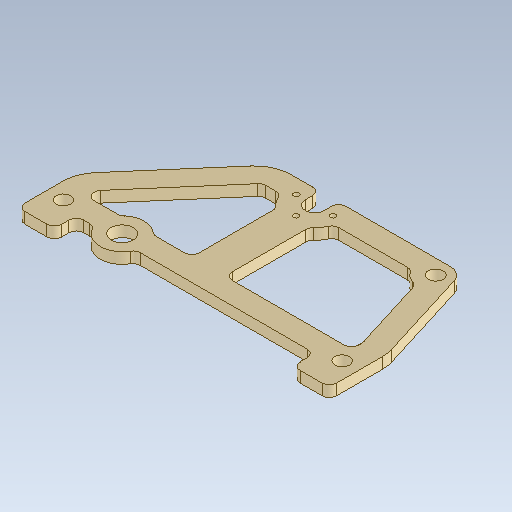
# Autodesk Inventor part: Опора катушки (врунтренняя)
Saved by Autodesk Inventor 2021.1 (Build 251245010, 245A)
## iProperties
Created: 2026-04-13
Part Number: Опора катушки (врунтренняя)
Material: Типовые
Document SubType Name: Modeling
Designer: Андрей Тарасов
Density: 1 g/cm^3
Appearance: По умолчанию
Author: Андрей Тарасов
Autodesk Inventor part; units mm, degrees
ref_plane "YZ Plane" through (0, 0, 0) normal (1, 0, 0) x (0, 1, 0)
ref_plane "XZ Plane" through (0, 0, 0) normal (0, 1, 0) x (-1, 0, 0)
ref_plane "XY Plane" through (0, 0, 0) normal (0, 0, 1) x (1, 0, 0)
sketch "Эскиз1" plane through (0, 0, 0) normal (0, 0, 1) x (1, 0, 0)
  circle A0 centre (0, 0) radius 60 construction
  line L0 (-80, -70) -> (-80, -50)
  line L1 (-80, -50) -> (-30, 8)
  line L2 (-30, 8) -> (72, 8)
  line L3 (72, 8) -> (90, -50)
  line L4 (90, -50) -> (90, -70)
  line L5 (90, -70) -> (-80, -70)
  line L6 (0, -110.4) -> (0, 88.4) construction
  line L7 (-115.4, 0) -> (132.4, 0) construction
  line L8 (-80, -50) -> (90, -50) construction
  circle A1 centre (67, -35) radius 12.5 construction
  circle A2 centre (0, 0) radius 5.1
  circle A3 centre (66, 0) radius 4.1
  circle A4 centre (67, -35) radius 4
  circle A5 centre (67, -35) radius 8.5 construction
  line L9 (67, -49.1463) -> (67, -22.5) construction
  circle A6 centre (67, -43.5) radius 1.6
  circle A7 centre (67, -26.5) radius 1.6
  line L10 (-24.5014, -4) -> (-68, -54.4584)
  line L11 (-68, -54.4584) -> (-68, -58)
  line L12 (-68, -58) -> (78, -58)
  line L13 (78, -58) -> (78, -51.8193)
  line L14 (78, -51.8193) -> (63.1595, -4)
  line L15 (63.1595, -4) -> (-24.5014, -4)
  arc A8 (-3.5925, -14.5634) -> (14.4568, -4) centre (0, 0) ccw
  arc A9 (-14.4568, -4) -> (-3.5925, -14.5634) centre (0, 0) ccw
  arc A10 (14.4568, -4) -> (-14.4568, -4) centre (0, 0) ccw construction
  line L16 (-9, -58) -> (-9, -12)
  line L17 (9, -58) -> (9, -12)
  arc A11 (65.0062, -9.9505) -> (56.8348, -4) centre (66, 0) ccw construction
  line L18 (68.4354, -21) -> (58.4354, -21)
  line L19 (58.4354, -21) -> (47.8258, -58)
  arc A12 (56.8348, -4) -> (65.0062, -9.9505) centre (66, 0) ccw
  line L20 (-80, -70) -> (-80, -82)
  line L21 (-80, -82) -> (-60, -82)
  line L22 (-60, -82) -> (-60, -70)
  line L23 (90, -70) -> (90, -82)
  line L24 (90, -82) -> (70, -82)
  line L25 (70, -82) -> (70, -70)
  circle A13 centre (-71, -66) radius 4
  circle A14 centre (81, -66) radius 4
  line L26 (-80, -66) -> (90, -66) construction
  line L27 (-5.1, 0) -> (-5.1, 8)
  line L28 (5.1, 0) -> (5.1, 8)
  circle A15 centre (37.4657, -40.2656) radius 6
  circle A16 centre (37.4657, -40.2656) radius 12
  circle A17 centre (67, -35) radius 30 construction
  circle A18 centre (0, 0) radius 55 construction
  line L29 (9, -40.2656) -> (74.4144, -40.2656) construction
  line L30 (9, -47.2656) -> (50.9039, -47.2656)
  line L31 (9, -33.2656) -> (54.9183, -33.2656)
  line L32 (69.7458, -32.0913) -> (70, -32.0913)
  circle A19 centre (0, 0) radius 10.05 construction
  circle A20 centre (-10.05, 0) radius 1.5
  circle A21 centre (10.05, 0) radius 1.5
  circle A22 centre (0, -10.05) radius 1.5
  circle A23 centre (-39, -66) radius 12
  circle A24 centre (-39, -66) radius 6
  point P0 (56.8348, -4)
  point P1 (65.0062, -9.9505)
  point P2 (59.5152, -7.6123)
  point P3 (27.7189, -33.2656)
  point P4 (27.7189, -47.2656)
  point P5 (47.2125, -47.2656)
  point P6 (47.2125, -33.2656)
  point P7 (3.1639, -4)
  point P8 (-3.1639, -4)
  point P9 (-27.6863, -70)
  point P10 (-50.3137, -70)
  point P11 (-30.0557, -58)
  point P12 (-47.9443, -58)
  dimension "d0" = 120
  dimension "d1" = 25
  dimension "d14" = 8
  dimension "d44" = 60
  dimension "d45" = 110
  dimension "d2" = 10.2
  dimension "d3" = 8
  dimension "d5" = 20
  dimension "d6" = 70
  dimension "d8" = 30
  dimension "d9" = 72
  dimension "d10" = 8.2
  dimension "d11" = 66
  dimension "d12" = 80
  dimension "d13" = 90
  dimension "d15" = 35
  dimension "d17" = 17
  dimension "d19" = 3.2
  dimension "d20" = 67
  dimension "d25" = 12
  dimension "d26" = 30
  dimension "d27" = 9
  dimension "d28" = 9
  dimension "d29" = 20
  dimension "d31" = 21
  dimension "d32" = 106
  dimension "d33" = 10
  dimension "d35" = 20
  dimension "d36" = 12
  dimension "d37" = 8
  dimension "d38" = 8
  dimension "d39" = 16
  dimension "d40" = 9
  dimension "d41" = 9
  dimension "d42" = 12
  dimension "d43" = 24
  dimension "d47" = 7
  dimension "d48" = 7
  dimension "d52" = 3
  dimension "d53" = 3
  dimension "d54" = 3
  dimension "d55" = 20.1
  dimension "d56" = 24
  dimension "d57" = 12
  dimension "d58" = 32
  constraints: 62 end point, 36 point on line, 20 centre point, 20 point on circle, 11 coincident, 7 perpendicular, 6 vertical, 4 horizontal, 4 parallel, 2 tangent, 1 collinear, 1 equal radius, 1 vertical alignment, 19 other
  measures "d2" diameter of A2
  measures "d3" distance between parallel lines of L2 L7
  measures "d5" distance between parallel lines of L5 L8
  measures "d6" distance between parallel lines of L5 L7
  measures "d8" distance from line of L6 L1.end
  measures "d9" distance from line of L2.end L6
  measures "d10" diameter of A3
  measures "d11" distance from line of L6 A3.centre
  measures "d12" distance between parallel lines of L6 L0
  measures "d13" distance between parallel lines of L4 L6
  measures "d15" distance from line of L5 point (67, -35)
  measures "d17" diameter of A5
  measures "d19" diameter of A6
  measures "d20" distance between parallel lines of L9 L6
  measures "d25" distance between parallel lines of L1 L10
  measures "d26" diameter of A8
  measures "d27" distance between parallel lines of L6 L16
  measures "d28" distance between parallel lines of L17 L6
  measures "d29" diameter of A11
  measures "d31" distance between parallel lines of L18 L7
  measures "d32" angle of L18 L19
  measures "d33" distance of L18.start L18.end
  measures "d35" distance of L20.end L21.end
  measures "d36" distance of L0.start L20.end
  measures "d37" diameter of A13
  measures "d38" diameter of A14
  measures "d39" distance between parallel lines of L21 L26
  measures "d40" distance from line of A13.centre L0
  measures "d41" distance from line of L4 A14.centre
  measures "d42" diameter of A15
  measures "d43" diameter of A16
  measures "d47" distance between parallel lines of L29 L30
  measures "d48" distance between parallel lines of L29 L31
  measures "d52" diameter of A20
  measures "d53" diameter of A21
  measures "d54" diameter of A22
  measures "d55" diameter of A19
  measures "d56" diameter of A23
  measures "d57" diameter of A24
  measures "d58" distance of A13.centre A23.centre
extrude "Выдавливание1" add sketch "Эскиз1" along normal blind 6 contours L0 L1 L2 L27 A2 L15 L10 L11 L12 A23 L5 | L5 L22 L21 L20 | A23 L12 L5 A24 | L5 A24 A23 | L2 L3 L4 L5 A23 L12 L13 L14 L15 A2 L28 | A23 L12 | A2 L15 A8 A9 | L5 L23 L24 L25 | L16 A9 A8 L17 L12 | L15 L14 A12
fillet "Сопряжение1" radius 4 24 edges at (9, -12, 3) (-24.5014, -4, 3) (-9, -58, 3) (-68, -54.4584, 3) (-68, -58, 3) (9, -58, 3) (56.8348, -4, 3) (65.0062, -9.9505, 3) (-80, -82, 3) (-60, -82, 3) (-60, -70, 3) (70, -70, 3) (70, -82, 3) (90, -82, 3) (5.1, 8, 3) (-5.1, 8, 3) (78, -58, 3) (-14.4568, -4, 3) (-9, -12, 3) (14.4568, -4, 3) (-47.9443, -58, 3) (-30.0557, -58, 3) (-50.3137, -70, 3) (-27.6863, -70, 3)
fillet "Сопряжение1" radius 20 3 edges at (-80, -50, 3) (-30, 8, 3) (90, -50, 3)
fillet "Сопряжение1" radius 8 2 edges at (72, 8, 3) (78, -51.8193, 3)
equation "\"d28\" = d27"
